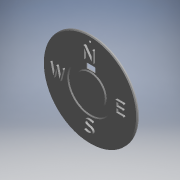
# Autodesk Inventor part: 風向
Saved by Autodesk Inventor 2021 (Build 250183000, 183)
## iProperties
Part Number: 風向
Material: 一般
Document SubType Name: 塑型
Designer: aura0
Appearance: 預設
Author: aura0
Autodesk Inventor part; units mm, degrees
ref_plane "YZ 平面" through (0, 0, 0) normal (1, 0, 0) x (0, 1, 0)
ref_plane "XZ 平面" through (0, 0, 0) normal (0, 1, 0) x (-1, 0, 0)
ref_plane "XY 平面" through (0, 0, 0) normal (0, 0, 1) x (1, 0, 0)
sketch "草圖1" plane through (0, 0, 0) normal (0, 0, 1) x (1, 0, 0)
  circle A0 centre (0, 0) radius 75
  dimension "d0" = 150
  constraints: 1 centre point, 1 coincident
  measures "d0" diameter of A0
extrude "擠出1" add sketch "草圖1" along normal blind 3
sketch "草圖2" plane through (0, 0, 3) normal (0, 0, 1) x (1, 0, 0)
  circle A0 centre (0, 0) radius 35
  circle A1 centre (0, 0) radius 25
  dimension "d3" = 70
  dimension "d4" = 50
  constraints: 2 centre point, 2 coincident
  measures "d3" diameter of A0
  measures "d4" diameter of A1
extrude "擠出2" cut sketch "草圖2" against normal blind 1.5
sketch "草圖3" plane through (0, 0, 1.5) normal (0, 0, 1) x (1, 0, 0)
  line L0 (-7, 26) -> (7, 26)
  line L1 (7, 26) -> (7, 34)
  line L2 (7, 34) -> (-7, 34)
  line L3 (-7, 34) -> (-7, 26)
  line L4 (-7, 26) -> (7, 34) construction
  line L5 (7, 26) -> (-7, 34) construction
  point P0 (0, 0)
  point P1 (0, 30)
  dimension "d7" = 14
  dimension "d8" = 8
  dimension "d9" = 30
  constraints: 12 end point, 2 midpoint, 2 parallel, 1 horizontal, 1 perpendicular
  measures "d7" distance of L2.end L1.end
  measures "d8" distance of L1.end L0.end
  measures "d9" distance of point (0, 0) point (0, 30)
extrude "擠出3" cut sketch "草圖3" against normal blind 1.5
sketch "草圖4" plane through (0, 0, 3) normal (0, 0, 1) x (1, 0, 0)
  circle A0 centre (0, 67) radius 1.65
  point P0 (0, 0)
  dimension "d12" = 67
  dimension "d13" = 3.3
  constraints: 1 centre point
  measures "d12" distance of point (0, 0) A0.centre
  measures "d13" diameter of A0
extrude "擠出4" cut sketch "草圖4" against normal through all
sketch "草圖5" plane through (0, 0, 3) normal (0, 0, 1) x (1, 0, 0)
  line L0 (-62.1661, 10.1549) -> (-38.5697, 10.1549) construction
  line L1 (-38.5697, 10.1549) -> (-38.5697, -10.6682) construction
  line L2 (-38.5697, -10.6682) -> (-62.1661, -10.6682) construction
  line L3 (-62.1661, -10.6682) -> (-62.1661, 10.1549) construction
  line L4 (39.8902, 10.0191) -> (57.8687, 10.0191) construction
  line L5 (57.8687, 10.0191) -> (57.8687, -9.7126) construction
  line L6 (57.8687, -9.7126) -> (39.8902, -9.7126) construction
  line L7 (39.8902, -9.7126) -> (39.8902, 10.0191) construction
  line L8 (-11.7628, 59.855) -> (10.8669, 59.855) construction
  line L9 (10.8669, 59.855) -> (10.8669, 39.855) construction
  line L10 (10.8669, 39.855) -> (-11.7628, 39.855) construction
  line L11 (-11.7628, 39.855) -> (-11.7628, 59.855) construction
  line L12 (-8.7979, -39.39) -> (8.5545, -39.39) construction
  line L13 (8.5545, -39.39) -> (8.5545, -59.6762) construction
  line L14 (8.5545, -59.6762) -> (-8.7979, -59.6762) construction
  line L15 (-8.7979, -59.6762) -> (-8.7979, -39.39) construction
  spline S0 degree 2 poles (-7.7556, 39.855) (-8.2923, 39.855) (-9.0615, 40.6063) (-9.0615, 41.143) knots 0 0 0 1 2 2 2
  line L16 (-9.0615, 41.143) -> (-9.0615, 57.9587)
  spline S1 degree 2 poles (-9.0615, 57.9587) (-9.0615, 58.728) (-7.9524, 59.855) (-7.2011, 59.855) knots 0 0 0 1 2 2 2
  line L17 (-7.2011, 59.855) -> (-6.8254, 59.855)
  spline S2 degree 2 poles (-6.8254, 59.855) (-5.9309, 59.855) (-5.2511, 59.0142) knots 0 0 0 1 1 1
  line L18 (-5.2511, 59.0142) -> (5.1424, 43.9874)
  spline S3 degree 2 poles (5.1424, 43.9874) (5.2855, 43.8264) (5.375, 43.8264) knots 0 0 0 1 1 1
  spline S4 degree 2 poles (5.375, 43.8264) (5.4286, 43.8264) (5.536, 43.9874) (5.536, 44.0947) knots 0 0 0 1 2 2 2
  line L19 (5.536, 44.0947) -> (5.536, 58.5312)
  spline S5 degree 2 poles (5.536, 58.5312) (5.536, 59.0679) (6.3052, 59.855) (6.8419, 59.855) knots 0 0 0 1 2 2 2
  spline S6 degree 2 poles (6.8419, 59.855) (7.3785, 59.855) (8.1657, 59.0679) (8.1657, 58.5312) knots 0 0 0 1 2 2 2
  line L20 (8.1657, 58.5312) -> (8.1657, 41.7154)
  spline S7 degree 2 poles (8.1657, 41.7154) (8.1657, 40.9462) (7.0387, 39.855) (6.2694, 39.855) knots 0 0 0 1 2 2 2
  line L21 (6.2694, 39.855) -> (5.9295, 39.855)
  spline S8 degree 2 poles (5.9295, 39.855) (5.4823, 39.855) (4.6594, 40.2664) (4.409, 40.6063) knots 0 0 0 1 2 2 2
  line L22 (4.409, 40.6063) -> (-6.0383, 55.7047)
  spline S9 degree 2 poles (-6.0383, 55.7047) (-6.1814, 55.8836) (-6.2708, 55.8836) knots 0 0 0 1 1 1
  spline S10 degree 2 poles (-6.2708, 55.8836) (-6.3245, 55.8836) (-6.4318, 55.7047) (-6.4318, 55.5974) knots 0 0 0 1 2 2 2
  line L23 (-6.4318, 55.5974) -> (-6.4318, 41.143)
  spline S11 degree 2 poles (-6.4318, 41.143) (-6.4318, 40.6063) (-7.2189, 39.855) (-7.7556, 39.855) knots 0 0 0 1 2 2 2
  spline S12 degree 2 poles (-55.7261, -9.8451) (-56.1912, -9.8451) (-56.8889, -9.1832) (-57.0677, -8.5571) knots 0 0 0 1 2 2 2
  line L24 (-57.0677, -8.5571) -> (-61.4864, 8.4017)
  spline S13 degree 2 poles (-61.4864, 8.4017) (-61.5579, 8.7416) (-61.5579, 8.9384) knots 0 0 0 1 1 1
  spline S14 degree 2 poles (-61.5579, 8.9384) (-61.5579, 9.4572) (-60.9676, 10.1549) (-60.5382, 10.1549) knots 0 0 0 1 2 2 2
  spline S15 degree 2 poles (-60.5382, 10.1549) (-60.1805, 10.1549) (-59.6259, 9.5824) (-59.5007, 9.1173) knots 0 0 0 1 2 2 2
  line L25 (-59.5007, 9.1173) -> (-55.905, -5.677)
  spline S16 degree 2 poles (-55.905, -5.677) (-55.8334, -5.9095) (-55.744, -5.9095) knots 0 0 0 1 1 1
  spline S17 degree 2 poles (-55.744, -5.9095) (-55.6545, -5.9095) (-55.583, -5.677) knots 0 0 0 1 1 1
  line L26 (-55.583, -5.677) -> (-51.9515, 9.0636)
  spline S18 degree 2 poles (-51.9515, 9.0636) (-51.8441, 9.5645) (-51.1644, 10.1549) (-50.7708, 10.1549) knots 0 0 0 1 2 2 2
  spline S19 degree 2 poles (-50.7708, 10.1549) (-50.3593, 10.1549) (-49.6796, 9.5645) (-49.5722, 9.0636) knots 0 0 0 1 2 2 2
  line L27 (-49.5722, 9.0636) -> (-45.9407, -5.677)
  spline S20 degree 2 poles (-45.9407, -5.677) (-45.8692, -5.9095) (-45.7797, -5.9095) knots 0 0 0 1 1 1
  spline S21 degree 2 poles (-45.7797, -5.9095) (-45.6903, -5.9095) (-45.6187, -5.677) knots 0 0 0 1 1 1
  line L28 (-45.6187, -5.677) -> (-42.023, 9.1173)
  spline S22 degree 2 poles (-42.023, 9.1173) (-41.8978, 9.5824) (-41.3432, 10.1549) (-40.9855, 10.1549) knots 0 0 0 1 2 2 2
  spline S23 degree 2 poles (-40.9855, 10.1549) (-40.5561, 10.1549) (-39.9658, 9.4572) (-39.9658, 8.9384) knots 0 0 0 1 2 2 2
  spline S24 degree 2 poles (-39.9658, 8.9384) (-39.9658, 8.7416) (-40.0373, 8.4017) knots 0 0 0 1 1 1
  line L29 (-40.0373, 8.4017) -> (-44.4559, -8.5571)
  spline S25 degree 2 poles (-44.4559, -8.5571) (-44.6348, -9.1832) (-45.3325, -9.8451) (-45.7976, -9.8451) knots 0 0 0 1 2 2 2
  spline S26 degree 2 poles (-45.7976, -9.8451) (-46.2806, -9.8451) (-47.0141, -9.1117) (-47.1572, -8.5571) knots 0 0 0 1 2 2 2
  line L30 (-47.1572, -8.5571) -> (-50.6098, 5.0744)
  spline S27 degree 2 poles (-50.6098, 5.0744) (-50.6813, 5.3069) (-50.7708, 5.3069) knots 0 0 0 1 1 1
  spline S28 degree 2 poles (-50.7708, 5.3069) (-50.8602, 5.3069) (-50.9139, 5.0744) knots 0 0 0 1 1 1
  line L31 (-50.9139, 5.0744) -> (-54.3665, -8.5571)
  spline S29 degree 2 poles (-54.3665, -8.5571) (-54.5096, -9.1117) (-55.2431, -9.8451) (-55.7261, -9.8451) knots 0 0 0 1 2 2 2
  spline S30 degree 2 poles (0.1288, -59.6762) (-3.449, -59.6762) (-6.5796, -58.3345) knots 0 0 0 1 1 1
  spline S31 degree 2 poles (-6.5796, -58.3345) (-6.9016, -58.1914) (-7.3846, -57.5116) (-7.3846, -57.1539) knots 0 0 0 1 2 2 2
  spline S32 degree 2 poles (-7.3846, -57.1539) (-7.3846, -56.6351) (-6.7048, -55.9374) (-6.204, -55.9374) knots 0 0 0 1 2 2 2
  spline S33 degree 2 poles (-6.204, -55.9374) (-5.8998, -55.9374) (-5.6673, -56.0447) knots 0 0 0 1 1 1
  spline S34 degree 2 poles (-5.6673, -56.0447) (-3.0555, -57.2075) (-0.1217, -57.2075) knots 0 0 0 1 1 1
  spline S35 degree 2 poles (-0.1217, -57.2075) (4.7799, -57.2075) (4.7799, -53.9875) knots 0 0 0 1 1 1
  spline S36 degree 2 poles (4.7799, -53.9875) (4.7799, -53.1467) (4.1717, -52.61) knots 0 0 0 1 1 1
  spline S37 degree 2 poles (4.1717, -52.61) (3.5993, -52.0734) (1.9177, -51.4472) (-0.0322, -50.9464) knots 0 0 0 1 2 2 2
  spline S38 degree 2 poles (-0.0322, -50.9464) (-2.2684, -50.3918) (-3.7174, -49.7836) knots 0 0 0 1 1 1
  spline S39 degree 2 poles (-3.7174, -49.7836) (-5.4526, -49.1396) (-7.1879, -46.7961) (-7.1879, -45.204) knots 0 0 0 1 2 2 2
  spline S40 degree 2 poles (-7.1879, -45.204) (-7.1879, -43.5939) (-6.3471, -42.2344) knots 0 0 0 1 1 1
  spline S41 degree 2 poles (-6.3471, -42.2344) (-5.4705, -40.8569) (-2.0716, -39.39) (0.1288, -39.39) knots 0 0 0 1 2 2 2
  spline S42 degree 2 poles (0.1288, -39.39) (3.2415, -39.39) (5.746, -40.3202) knots 0 0 0 1 1 1
  spline S43 degree 2 poles (5.746, -40.3202) (6.551, -40.6243) (6.551, -41.483) knots 0 0 0 1 1 1
  spline S44 degree 2 poles (6.551, -41.483) (6.551, -41.9303) (5.8891, -42.6816) (5.4061, -42.6816) knots 0 0 0 1 2 2 2
  spline S45 degree 2 poles (5.4061, -42.6816) (5.2093, -42.6816) (4.9588, -42.5743) knots 0 0 0 1 1 1
  spline S46 degree 2 poles (4.9588, -42.5743) (2.7585, -41.8229) (0.415, -41.8229) knots 0 0 0 1 1 1
  spline S47 degree 2 poles (0.415, -41.8229) (-1.839, -41.8229) (-4.576, -43.5045) (-4.576, -45.0072) knots 0 0 0 1 2 2 2
  spline S48 degree 2 poles (-4.576, -45.0072) (-4.576, -46.009) (-3.8963, -46.5993) knots 0 0 0 1 1 1
  spline S49 degree 2 poles (-3.8963, -46.5993) (-3.2701, -47.2075) (-1.4097, -47.9231) (0.4508, -48.3524) knots 0 0 0 1 2 2 2
  spline S50 degree 2 poles (0.4508, -48.3524) (2.8121, -48.9249) (4.0465, -49.4258) knots 0 0 0 1 1 1
  spline S51 degree 2 poles (4.0465, -49.4258) (5.5492, -49.9803) (7.3739, -52.3596) (7.3739, -54.1664) knots 0 0 0 1 2 2 2
  spline S52 degree 2 poles (7.3739, -54.1664) (7.3739, -55.7048) (6.4794, -57.0108) knots 0 0 0 1 1 1
  spline S53 degree 2 poles (6.4794, -57.0108) (5.5492, -58.2988) (2.2397, -59.6762) (0.1288, -59.6762) knots 0 0 0 1 2 2 2
  spline S54 degree 2 poles (43.8973, -9.7126) (43.3606, -9.7126) (42.5914, -8.9434) (42.5914, -8.4067) knots 0 0 0 1 2 2 2
  line L32 (42.5914, -8.4067) -> (42.5914, 8.6953)
  spline S55 degree 2 poles (42.5914, 8.6953) (42.5914, 9.2319) (43.3606, 10.0191) (43.8973, 10.0191) knots 0 0 0 1 2 2 2
  line L33 (43.8973, 10.0191) -> (55.1853, 10.0191)
  spline S56 degree 2 poles (55.1853, 10.0191) (55.7041, 10.0191) (56.4376, 9.2856) (56.4376, 8.7847) knots 0 0 0 1 2 2 2
  spline S57 degree 2 poles (56.4376, 8.7847) (56.4376, 8.2659) (55.7041, 7.5683) (55.1853, 7.5683) knots 0 0 0 1 2 2 2
  line L34 (55.1853, 7.5683) -> (45.561, 7.5683)
  spline S58 degree 2 poles (45.561, 7.5683) (45.2211, 7.5683) (45.2211, 7.2284) knots 0 0 0 1 1 1
  line L35 (45.2211, 7.2284) -> (45.2211, 1.3965)
  line L36 (45.2211, 1.3965) -> (54.1835, 1.3965)
  spline S59 degree 2 poles (54.1835, 1.3965) (54.6844, 1.3965) (55.4179, 0.6631) (55.4179, 0.1622) knots 0 0 0 1 2 2 2
  spline S60 degree 2 poles (55.4179, 0.1622) (55.4179, -0.3566) (54.6844, -1.0543) (54.1835, -1.0543) knots 0 0 0 1 2 2 2
  line L37 (54.1835, -1.0543) -> (45.2211, -1.0543)
  line L38 (45.2211, -1.0543) -> (45.2211, -6.9219)
  spline S61 degree 2 poles (45.2211, -6.9219) (45.2211, -7.2618) (45.561, -7.2618) knots 0 0 0 1 1 1
  line L39 (45.561, -7.2618) -> (55.1853, -7.2618)
  spline S62 degree 2 poles (55.1853, -7.2618) (55.7041, -7.2618) (56.4376, -7.9774) (56.4376, -8.4961) knots 0 0 0 1 2 2 2
  spline S63 degree 2 poles (56.4376, -8.4961) (56.4376, -8.997) (55.7041, -9.7126) (55.1853, -9.7126) knots 0 0 0 1 2 2 2
  line L40 (55.1853, -9.7126) -> (43.8973, -9.7126)
  point P0 (0, 0)
  constraints: 8 other
extrude "擠出5" add sketch "草圖5" along normal blind 3
chamfer "倒角1" distance 1.25 angle 45 3 edges at (-25, 0, 3) (-35, 0, 3) (-75, 0, 3)
